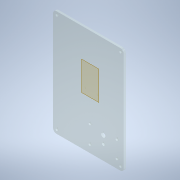
# Autodesk Inventor part: TopPlate
Saved by Autodesk Inventor 2021 (Build 250183000, 183)
## iProperties
Created: 2020-09-18
Part Number: TopPlate
Material: Glass
Document SubType Name: Modeling
Designer: siwat
Density: 2.18 g/cm^3
Appearance: Clear
Author: siwat
Autodesk Inventor part; units mm, degrees
ref_plane "YZ Plane" through (0, 0, 0) normal (1, 0, 0) x (0, 1, 0)
ref_plane "XZ Plane" through (0, 0, 0) normal (0, 1, 0) x (-1, 0, 0)
ref_plane "XY Plane" through (0, 0, 0) normal (0, 0, 1) x (1, 0, 0)
ref_plane "Work Plane1" through (0, 0, 0) normal (0, 0, 1) x (1, 0, 0)
sketch "Sketch1" plane through (0, 0, 0) normal (0, 0, 1) x (1, 0, 0)
  line L0 (39.3474, 50.6868) -> (-50.6526, 50.6868)
  line L1 (-55.6526, 45.6868) -> (-55.6526, -94.3132)
  line L2 (-50.6526, -99.3132) -> (39.3474, -99.3132)
  line L3 (44.3474, -94.3132) -> (44.3474, 45.6868)
  circle A0 centre (15.3748, -79.3757) radius 5.0406
  circle A1 centre (15.3748, -68.2846) radius 2.0418
  arc A2 (44.3474, 45.6868) -> (39.3474, 50.6868) centre (39.3474, 45.6868) ccw
  arc A3 (39.3474, -99.3132) -> (44.3474, -94.3132) centre (39.3474, -94.3132) ccw
  arc A4 (-55.6526, -94.3132) -> (-50.6526, -99.3132) centre (-50.6526, -94.3132) ccw
  arc A5 (-50.6526, 50.6868) -> (-55.6526, 45.6868) centre (-50.6526, 45.6868) ccw
  circle A6 centre (39.3474, 45.6868) radius 1.5
  circle A7 centre (39.3474, -94.3132) radius 1.5
  circle A8 centre (-50.6526, -94.3132) radius 1.5
  circle A9 centre (-50.6526, 45.6868) radius 1.5
  circle A10 centre (-4.0059, -64.1251) radius 1.5
  circle A11 centre (-4.0059, -89.321) radius 1.5
  circle A12 centre (34.2474, -64.1251) radius 1.5
  circle A13 centre (34.2474, -87.7789) radius 1.5
  point P0 (0, 0)
  point P1 (15.2639, -84.621)
  point P2 (44.3474, 50.6868)
  point P3 (-55.6526, -99.3132)
  point P4 (44.3474, -99.3132)
  dimension "d0" = 100
  dimension "d1" = 150
  dimension "d2" = 5
  dimension "d3" = 3
  dimension "d4" = 3
  dimension "d5" = 3
  dimension "d6" = 3
  dimension "d7" = 3
  dimension "d8" = 3
  dimension "d9" = 3
  dimension "d10" = 3
  constraints: 14 centre point, 8 end point, 8 point on circle, 8 tangent, 6 point on line, 4 coincident, 3 equal radius, 2 parallel, 1 perpendicular
  measures "d0" distance of point (-55.653, -99.313) point (44.347, -99.313)
  measures "d1" distance of point (44.347, -99.313) point (44.347, 50.687)
  measures "d2" radius of A2
  measures "d3" diameter of A6
  measures "d4" diameter of A7
  measures "d5" diameter of A8
  measures "d6" diameter of A9
  measures "d7" diameter of A10
  measures "d8" diameter of A11
  measures "d9" diameter of A12
  measures "d10" diameter of A13
extrude "Extrusion1" add sketch "Sketch1" along normal blind 3
sketch "Sketch2" plane through (0, 0, 0) normal (0, 0, -1) x (-1, 0, 0)
  circle A0 centre (-6.6801, -58.8323) radius 1.4403
  circle A1 centre (-24.0209, -58.8323) radius 1.4576
  point P0 (0, 0)
  constraints: 2 centre point
extrude "Extrusion2" add sketch "Sketch2" along normal blind 1.5
body "Solid1"
